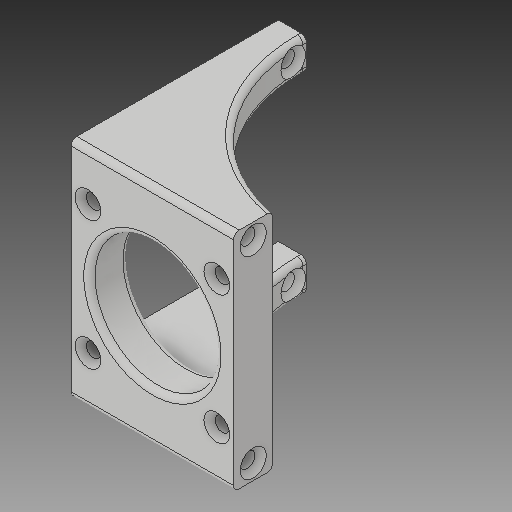
# Autodesk Inventor part: Nema11_holder
Saved by Autodesk Inventor 2019 (Build 230136000, 136)
## iProperties
Created: 2021-10-13
Part Number: Nema11_holder
Material: Generic
Document SubType Name: Modeling
Designer: Pokick
Density: 1 g/cm^3
Appearance: Default
Author: Pokick
Autodesk Inventor part; units mm, degrees
ref_plane "YZ Plane" through (0, 0, 0) normal (1, 0, 0) x (0, 1, 0)
ref_plane "XZ Plane" through (0, 0, 0) normal (0, 1, 0) x (-1, 0, 0)
ref_plane "XY Plane" through (0, 0, 0) normal (0, 0, 1) x (1, 0, 0)
sketch "Sketch1" plane through (0, 0, 0) normal (0, 0, 1) x (1, 0, 0)
  line L0 (11.5, -11.5) -> (-11.5, -11.5) construction
  line L1 (-11.5, -11.5) -> (-11.5, 11.5) construction
  line L2 (-11.5, 11.5) -> (11.5, 11.5) construction
  line L3 (11.5, 11.5) -> (11.5, -11.5) construction
  line L4 (11.5, -11.5) -> (-11.5, 11.5) construction
  line L5 (-11.5, -11.5) -> (11.5, 11.5) construction
  line L6 (14.5, -20) -> (-14.5, -20)
  line L7 (-14.5, -20) -> (-14.5, 20)
  line L8 (-14.5, 20) -> (14.5, 20)
  line L9 (14.5, 20) -> (14.5, -20)
  line L10 (14.5, -20) -> (-14.5, 20) construction
  line L11 (-14.5, -20) -> (14.5, 20) construction
  circle A0 centre (0, 0) radius 11.25
  circle A1 centre (11.5, 11.5) radius 1.3
  circle A2 centre (11.5, -11.5) radius 1.3
  circle A3 centre (-11.5, -11.5) radius 1.3
  circle A4 centre (-11.5, 11.5) radius 1.3
  dimension "d0" = 23
  dimension "d1" = 23
  dimension "d2" = 29
  dimension "d3" = 40
  dimension "d4" = 22.5
  dimension "d5" = 2.6
  dimension "d6" = 2.6
  dimension "d7" = 2.6
  dimension "d8" = 2.6
  constraints: 24 end point, 5 centre point, 5 coincident, 4 midpoint, 4 parallel, 2 horizontal, 2 perpendicular
  measures "d0" distance of L1.end L2.end
  measures "d1" distance of L0.end L1.end
  measures "d2" distance of L7.end L8.end
  measures "d3" distance of L6.end L7.end
  measures "d4" diameter of A0
  measures "d5" diameter of A1
  measures "d6" diameter of A2
  measures "d7" diameter of A3
  measures "d8" diameter of A4
extrude "Extrusion1" add sketch "Sketch1" along normal blind 7
sketch "Sketch2" plane through (0, 0, 0) normal (0, 0, -1) x (-1, 0, 0)
  line L0 (-14.5, 20) -> (14.5, 20) construction
  line L1 (-14.5, -20) -> (14.5, -20) construction
  line L2 (14.5, -20) -> (14.5, 20) construction
  line L3 (14.5, 20) -> (-14.5, 20) construction
  line L4 (-14.5, 20) -> (-14.5, -20) construction
  line L5 (-14.5, -20) -> (14.5, 20) construction
  line L6 (14.5, -20) -> (-14.5, 20) construction
  line L7 (14.5, 20) -> (9.5, 20)
  line L8 (9.5, 20) -> (9.5, -20)
  line L9 (9.5, -20) -> (14.5, -20)
  line L10 (14.5, -20) -> (14.5, 20)
  line L11 (-14.25, -14.25) -> (14.25, -14.25) construction
  line L12 (14.25, -14.25) -> (14.25, 14.25) construction
  line L13 (14.25, 14.25) -> (-14.25, 14.25) construction
  line L14 (-14.25, 14.25) -> (-14.25, -14.25) construction
  line L15 (-14.25, -14.25) -> (14.25, 14.25) construction
  line L16 (14.25, -14.25) -> (-14.25, 14.25) construction
  line L17 (9.5, 14.25) -> (14.5, 14.25)
  line L18 (14.5, -20) -> (14.5, 20) projected
  line L19 (9.5, -14.25) -> (14.5, -14.25)
  point P0 (0, 0)
  dimension "d11" = 5
  dimension "d12" = 40
  dimension "d13" = 28.5
  dimension "d14" = 28.5
  constraints: 36 end point, 7 point on line, 6 parallel, 4 horizontal, 4 midpoint, 3 perpendicular
  measures "d11" distance of L9.end L8.end
  measures "d12" distance of L8.end L7.end
  measures "d13" distance of L13.end L12.end
  measures "d14" distance of L12.end L11.end
extrude "Extrusion2" add sketch "Sketch2" along normal blind 30 contours L10 L17 L8 L7 | L10 L9 L8 L19
fillet "Fillet1" radius 30 2 edges at (-9.5, 17.125, 0) (-9.5, -17.125, 0)
sketch "Sketch3" plane through (-14.5, -20, 7) normal (-1, 0, 0) x (0, 0, 1)
  line L0 (-7, 20) -> (-19, 20) construction
  line L1 (-36.3939, 0) -> (-36.3939, 5.75) construction
  line L2 (-34.5, 2.75) -> (-3.5, 2.75) construction
  line L3 (-3.5, 2.75) -> (-3.5, 37.25) construction
  line L4 (-3.5, 37.25) -> (-34.5, 37.25) construction
  line L5 (-34.5, 37.25) -> (-34.5, 2.75) construction
  line L6 (-34.5, 2.75) -> (-3.5, 37.25) construction
  line L7 (-3.5, 2.75) -> (-34.5, 37.25) construction
  circle A0 centre (-34.5, 2.75) radius 1.35
  circle A1 centre (-34.5, 37.25) radius 1.35
  circle A2 centre (-3.5, 2.75) radius 1.35
  circle A3 centre (-3.5, 37.25) radius 1.35
  dimension "d18" = 12
  dimension "d19" = 31
  dimension "d20" = 34.5
  dimension "d21" = 2.7
  dimension "d22" = 2.7
  dimension "d23" = 2.7
  dimension "d24" = 2.7
  constraints: 14 end point, 4 centre point, 4 coincident, 2 midpoint, 2 parallel, 2 perpendicular, 1 horizontal
  measures "d18" distance of L0.start L0.end
  measures "d19" distance of L4.end L3.end
  measures "d20" distance of L3.end L2.end
  measures "d21" diameter of A0
  measures "d22" diameter of A1
  measures "d23" diameter of A2
  measures "d24" diameter of A3
extrude "Extrusion3" cut sketch "Sketch3" against normal blind 30
chamfer "Chamfer1" distance 1 angle 45 4 edges at (-9.4951, -17.2488, -28.85) (-9.4951, 17.2512, -28.85) (14.5, 17.25, 2.15) (14.5, -17.25, 2.15)
chamfer "Chamfer2" distance 1 angle 45 4 edges at (10.2, -11.5, 7) (-12.8, -11.5, 7) (10.2, 11.5, 7) (-12.8, 11.5, 7)
fillet "Fillet2" radius 1 1 edges at (-11.25, 0, 7)
fillet "Fillet3" radius 1 1 edges at (-11.25, 0, 0)
fillet "Fillet4" radius 1 10 edges at (0, -20, 7) (0, 20, 7) (-9.5, 20, -29.6969) (-2.7379, 20, -10.4202) (-9.5, -20, -29.6969) (-2.7379, -20, -10.4202) (-9.5, -14.25, -29.6969) (-2.7379, -14.25, -10.4202) (-9.5, 14.25, -29.6969) (-2.7379, 14.25, -10.4202)
body "Solid1"
